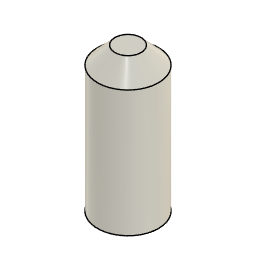
Joystick v2 (Autodesk Fusion 360 design; units mm, degrees)
Autodesk Fusion 360 part; units mm, degrees
note: some values were not read from the file. Set by a fixed rule: which face or edge a step refers to.
sketch "Sketch1" plane through (0, 0, 0) normal (0, 0, 1) x (1, 0, 0)
  circle A0 centre (0, 0) radius 3.5
  circle A1 centre (0, 0) radius 2
  line L0 (-1.5, 1.3229) -> (-1.5, -1.3229)
  line L1 (1.5, -1.3229) -> (1.5, 1.3229)
  dimension "d1" = 4
  dimension "d2" = 7
  dimension "d3" = 3
  constraint coincident A0.centre A1.centre
  constraint coincident A1 L0.start
  constraint coincident A1 L0.end
  constraint vertical L0
  constraint coincident A1 L1.start
  constraint coincident A1 L1.end
  constraint parallel L0 L1
  constraint equal L0 L1
  measures "d1" diameter of A1
  measures "d2" diameter of A0
  measures "d3" distance of L0 L1
extrude "Extrude1" add sketch "Sketch1" along normal blind 4.5 contours A0 | A1 L1 | A1 L0
extrude "Extrude2" add sketch "Sketch1" against normal blind 1.5
extrude "Extrude3" add sketch "Sketch1" along normal blind 4.5 and the other way blind -15 contours A0 | A1 L1 | A1 L0 L1 | A1 L0
move_face "OffsetFaces1" offset -0.1 7 faces at (1.562, 1.2491, -1) (-1.3689, 1.4581, -1) (-1.9422, -0.4772, -1) (1.2256, -1.5805, -1) (1.562, -1.2491, -0.5) (-1.436, 1.3921, 3) (1.2256, -1.5805, 3)
move_face "OffsetFaces2" offset -0.1 2 faces at (1.5, 0.4899, 1.5) (-1.5, -0.4899, 1.5)
chamfer "Chamfer2" distance 2 angle 45 1 edges at (-3.2631, -1.2657, 15)
sketch "Sketch2" plane through (0, 0, 0) normal (0, 1, 0) x (1, 0, 0)
  arc A0 (5.7403, -16.1418) -> (-5.7403, -16.1418) centre (0, -30) ccw
  line L0 (0, -30) -> (-5.7403, -16.1418)
  line L1 (0, -30) -> (5.7403, -16.1418)
  line L2 (0, -15) -> (0, 0)
  line L3 (0, -15) -> (0, -30)
  line L4 (-3.5, -15) -> (3.5, -15)
  arc A1 (6.1229, -15.2179) -> (-6.1229, -15.2179) centre (0, -30) ccw
  line L5 (-6.1229, -15.2179) -> (-5.7403, -16.1418)
  line L6 (6.1229, -15.2179) -> (5.7403, -16.1418)
  dimension "d14" = 45
  dimension "d15" = 15
  dimension "d16" = 1
  constraint coincident A0.centre L0.start
  constraint midpoint A0 L2.start
  constraint coincident L2.end origin
  constraint vertical L2
  constraint vertical L3
  constraint tangent A0 L4
  constraint parallel L0 L5
  constraint parallel L1 L6
  measures "d14" angle of L0 L1
  measures "d15" radius of A0
revolve "Revolve1" [rolled back] along angle 360
chamfer "Chamfer1" [rolled back] distance 1
